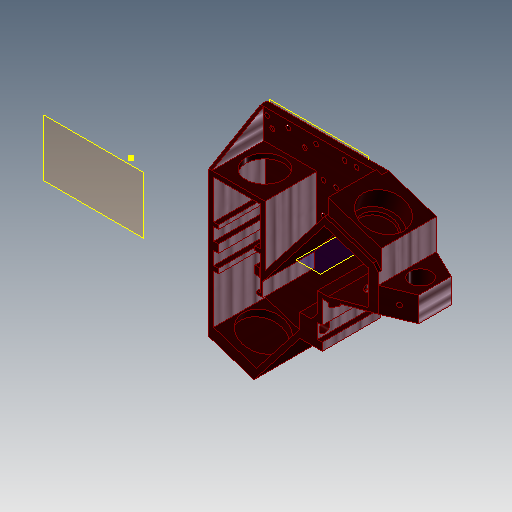
# Autodesk Inventor part: cellSTORM_v5_opticalstage
Saved by Autodesk Inventor 2019.4 (Build 234330000, 330)
## iProperties
Created: 2020-04-25
Part Number: cellSTORM_v5_opticalstage
Material: Generic
Document SubType Name: Modeling
Designer: diederichbenedict
Density: 1 g/cm^3
Appearance: Red
Author: diederichbenedict
Autodesk Inventor part; units mm, degrees
ref_plane "YZ Plane" through (0, 0, 0) normal (1, 0, 0) x (0, 1, 0)
ref_plane "XZ Plane" through (0, 0, 0) normal (0, 1, 0) x (-1, 0, 0)
ref_plane "XY Plane" through (0, 0, 0) normal (0, 0, 1) x (1, 0, 0)
ref_plane "Work Plane1" through (0, 0, 0) normal (0, 0, 1) x (1, 0, 0)
ref_plane "Work Plane2" through (79.8747, 18.953, -59.1152) normal (0, 0, 1) x (1, 0, 0)
sketch "Sketch2" plane through (79.8747, 18.953, -59.1152) normal (0, 0, 1) x (1, 0, 0)
  line L0 (-28, -14.1495) -> (28, -14.1495) projected
  line L1 (28, -14.1495) -> (28, -9.1495) projected
  line L2 (28, -9.1495) -> (22, -9.1495) projected
  line L3 (22, -9.1495) -> (22, 17.8293) projected
  line L4 (22, 17.8293) -> (-22, 17.8293) projected
  line L5 (-22, 17.8293) -> (-22, -9.1495) projected
  line L6 (-22, -9.1495) -> (-28, -9.1495) projected
  line L7 (-28, -9.1495) -> (-28, -14.1495) projected
  line L8 (-28, -14.1495) -> (-32, -14.1495)
  line L9 (-28, -14.1495) -> (-24, -14.1495) construction
  line L10 (-32, -14.1495) -> (-32, -90.2028)
  line L11 (-32, -90.2028) -> (-4.0389, -99.2879)
  line L12 (-4.0389, -99.2879) -> (46.0734, -35.147)
  line L13 (46.0734, -35.147) -> (72.5683, -35.147)
  line L14 (72.5683, -35.147) -> (72.5683, 8.2211)
  line L15 (72.5683, 8.2211) -> (42.9972, 17.8293)
  line L16 (42.9972, 17.8293) -> (22, 17.8293)
  line L17 (-28.3388, -86.702) -> (-4.6575, -94.3965) projected
  line L18 (-4.3425, -94.236) -> (-28.4993, -86.387) projected
  line L19 (45.4114, 13.8905) -> (69.5683, 6.0415) projected
  line L20 (-27.6911, -86.6496) -> (-26.7997, -83.9062)
  line L21 (-3.5343, -94.4986) -> (-2.6429, -91.7552)
  line L22 (53.5499, -4.91) -> (-11.1218, -87.6859)
  line L23 (-22, 17.8293) -> (-32, 17.8293)
  line L24 (-32, 17.8293) -> (-32, -14.1495)
  point P0 (-79.8747, -18.953)
  point P1 (-26.7997, -83.9062)
  point P2 (-2.6429, -91.7552)
  dimension "d0" = 4
  dimension "d1" = 180
  dimension "d2" = 3
  dimension "d3" = 3
  dimension "d4" = 3
  dimension "d5" = 1
  constraints: 28 end point, 7 parallel, 3 collinear, 3 horizontal, 1 perpendicular, 7 other
  measures "d0" distance of L0.start L8.end
  measures "d1" angle of L8 L9
  measures "d2" distance between parallel lines of L19 L15
  measures "d3" distance from line of L19.end L14
  measures "d4" distance from line of L20 L10.end
  measures "d5" distance from line of L11.end L21
extrude "Extrusion1" add sketch "Sketch2" along normal blind 4
sketch "Sketch3" plane through (79.8747, 18.953, -55.1152) normal (0, 0, 1) x (1, 0, 0)
  line L0 (42.9972, 17.8293) -> (-32, 17.8293) projected
  line L1 (-32, 17.8293) -> (-32, -90.2028) projected
  line L2 (-32, -90.2028) -> (-4.0389, -99.2879) projected
  line L3 (-4.0389, -99.2879) -> (46.0734, -35.147) projected
  line L4 (46.0734, -35.147) -> (72.5683, -35.147) projected
  line L5 (72.5683, -35.147) -> (72.5683, 8.2211) projected
  line L6 (72.5683, 8.2211) -> (42.9972, 17.8293) projected
  line L7 (-27.1008, 14.8293) -> (42.5221, 14.8293)
  line L8 (42.5221, 14.8293) -> (69.5683, 6.0415)
  line L9 (66.4162, -32.147) -> (35.0734, -32.147)
  line L10 (-2.489, -92.4313) -> (-29, -83.8173)
  line L11 (-28.6512, -0.5207) -> (-0.8512, -0.5207) projected
  line L12 (-29, -3.5207) -> (-27.1008, -3.5207)
  line L13 (2.7488, -0.5207) -> (2.7488, -4.5207)
  line L14 (-0.2512, -3.5207) -> (-29, -3.5207)
  line L15 (-32, 17.8293) -> (-32, -90.2028) projected
  line L16 (-12.2512, -81.0102) -> (-12.2512, 6.7293) construction
  line L17 (52.4205, 1.7657) -> (-12.2512, -81.0102) construction
  line L18 (2.7488, -4.5207) -> (2.7488, -37.447)
  line L19 (2.7488, -37.447) -> (39.6078, 9.7303)
  line L20 (43.8723, 8.3447) -> (67.5537, 0.6501) projected
  line L21 (-0.2512, -3.5207) -> (-0.2512, -46.1597)
  line L22 (-0.2512, -46.1597) -> (39.3735, 4.5576)
  line L23 (39.3735, 4.5576) -> (66.4162, -4.2291)
  line L24 (39.6078, 9.7303) -> (69.5683, -0.0045)
  line L25 (-29, -83.8173) -> (-29, -3.5207)
  line L26 (69.5683, -0.0045) -> (72.5683, -3.7292)
  line L27 (72.5683, -35.147) -> (72.5683, 8.2211) projected
  line L28 (66.0925, 1.3476) -> (69.5683, -0.0045)
  line L29 (66.4162, -4.2291) -> (66.4162, -32.147)
  line L30 (-3.2512, -3.2707) -> (-3.2512, -19.4707) construction
  line L31 (-29.0012, -37.7707) -> (-0.5012, -37.7707) projected
  line L32 (-0.5012, -37.7707) -> (-0.5012, -30.5207) projected
  line L33 (-29.0012, -30.5207) -> (-0.5012, -30.5207) projected
  line L34 (-29.0012, -37.7707) -> (-29.0012, -30.5207) projected
  line L35 (-29.0012, -37.7707) -> (-0.5012, -37.7707) construction
  line L36 (-29, -37.7707) -> (-26, -37.7707) construction
  line L37 (-26, -37.7707) -> (-26, -42.7707) construction
  line L38 (-26, -42.7707) -> (-29, -42.7707) construction
  line L39 (-29, -42.7707) -> (-29, -37.7707) construction
  line L40 (-29, -42.7707) -> (-26, -42.7707)
  line L41 (-26, -42.7707) -> (-26, -37.7707)
  line L42 (-26, -37.7707) -> (-29, -37.7707)
  line L43 (-29, -37.7707) -> (-29, -42.7707)
  line L44 (-0.5012, -37.7707) -> (-3.5012, -37.7707)
  line L45 (-3.5012, -37.7707) -> (-3.5012, -42.7707)
  line L46 (-3.5012, -42.7707) -> (-0.5012, -42.7707)
  line L47 (-0.5012, -42.7707) -> (-0.5012, -37.7707)
  line L48 (-29, -27.5207) -> (-26, -27.5207)
  line L49 (-26, -27.5207) -> (-26, -30.0207)
  line L50 (-26, -30.0207) -> (-29, -30.0207)
  line L51 (-29, -30.0207) -> (-29, -27.5207)
  line L52 (-0.2512, -27.5207) -> (-3.5012, -27.5207)
  line L53 (-3.5012, -27.5207) -> (-3.5012, -30.0207)
  line L54 (-3.5012, -30.0207) -> (-0.2512, -30.0207)
  line L55 (-0.2512, -30.0207) -> (-0.2512, -27.5207)
  line L56 (-4.0389, -99.2879) -> (46.0734, -35.147) projected
  line L57 (46.0734, -35.147) -> (72.5683, -35.147) projected
  line L58 (39.6078, 9.7303) -> (45.1198, 17.1396)
  line L59 (72.5683, 8.2211) -> (42.9972, 17.8293) projected
  line L60 (72.5683, -3.7292) -> (72.5683, 8.2211)
  line L61 (72.5683, 8.2211) -> (45.1198, 17.1396)
  line L62 (2.7488, -0.5207) -> (-32, -0.5207)
  line L63 (35.0734, -32.147) -> (35.0734, -44.3536)
  line L64 (35.0734, -44.3536) -> (-2.489, -92.4313)
  line L65 (38.0734, -45.3866) -> (38.0734, -35.147)
  line L66 (38.0734, -35.147) -> (46.0734, -35.147)
  line L67 (38.0734, -45.3866) -> (42.0734, -45.3866)
  line L68 (42.0734, -45.3866) -> (42.0734, -48.3866)
  line L69 (42.0734, -48.3866) -> (35.7295, -48.3866)
  point P0 (-79.8747, -18.953)
  point P1 (-0.8512, -0.5207)
  point P2 (-32, -3.2707)
  dimension "d10" = 4
  dimension "d11" = 3
  dimension "d13" = 3
  dimension "d16" = 12
  dimension "d17" = 3
  dimension "d18" = 3
  dimension "d19" = 5
  dimension "d20" = 3
  dimension "d21" = 2.5
  dimension "d22" = 0.5
  dimension "d23" = 3
  dimension "d24" = 7
  dimension "d25" = 3
  dimension "d47" = 3
  dimension "d48" = 3
  dimension "d49" = 3
  dimension "d50" = 8
  dimension "d51" = 3
  dimension "d66" = 4
  constraints: 100 end point, 17 parallel, 15 point on line, 10 perpendicular, 8 horizontal, 6 vertical, 2 collinear, 13 other
  measures "d10" distance of L13.start L13.end
  measures "d13" distance between parallel lines of L22 L19
  measures "d16" distance between parallel lines of L22 L17
  measures "d18" distance of L37.end L38.end
  measures "d19" distance of L36.end L37.end
  measures "d20" distance of L46.end L45.end
  measures "d21" distance of L48.end L49.end
  measures "d22" distance between parallel lines of L33 L50
  measures "d24" distance between parallel lines of L2 L10
  measures "d25" distance between parallel lines of L25 L1
  measures "d47" distance between parallel lines of L9 L4
  measures "d48" distance between parallel lines of L64 L3
  measures "d49" distance between parallel lines of L63 L65
  measures "d50" distance from line of L3.end L65
  measures "d51" distance of L67.end L68.end
  measures "d66" distance between parallel lines of L68 L65
extrude "Extrusion2" add sketch "Sketch3" along normal blind 32 contours L62 L11 L13 L18 L19 L24 L20 L26 L5 L4 L66 L65 L3 L2 L1 | L54 L53 L52 L21 | L25 L31 L41 L40 | L25 L48 L49 L50 | L31 L47 L46 L45
ref_plane "Work Plane3" through (51.6835, -64.2382, -58.0722) normal (0.309017, 0.9510565, 0) x (-0.6726294, 0.2185505, 0.7069691)
ref_plane "Work Plane4" through (49.8294, -69.9446, -58.0722) normal (-0.309017, -0.9510565, 0) x (0.6723676, -0.2184655, 0.7072444)
sketch "Sketch7" plane through (50.8747, -64.8644, -23.1152) normal (0.309017, 0.9510565, 0) x (0.9510565, -0.309017, 0)
  circle A0 centre (13.9703, 17.35) radius 12.7 projected
  circle A1 centre (13.9703, 17.35) radius 13
  point P0 (-68.4289, -23.1152)
  dimension "d33" = 26
  constraints: 1 centre point, 1 coincident
  measures "d33" diameter of A1
extrude "Extrusion5" cut sketch "Sketch7" against normal up to surface (6 mm away) from surface at 0.8454 contours A0 | A1
sketch "Sketch8" plane through (79.8747, 18.953, -55.1152) normal (0, 0, 1) x (1, 0, 0)
  line L0 (-32, -90.2028) -> (-4.0389, -99.2879) projected
  line L1 (72.5683, -35.147) -> (72.5683, -3.7292) projected
  line L2 (69.5683, -0.0045) -> (39.6078, 9.7303) projected
  line L3 (39.6078, 9.7303) -> (2.7488, -37.447) projected
  line L4 (2.7488, -37.447) -> (2.7488, -0.5207) projected
  line L5 (-32, -0.5207) -> (-32, -90.2028) projected
  line L6 (-29, -30.5207) -> (-29, -30.0207) projected
  line L7 (-29, -30.0207) -> (-26, -30.0207) projected
  line L8 (-26, -30.0207) -> (-26, -27.5207) projected
  line L9 (-26, -27.5207) -> (-29, -27.5207) projected
  line L10 (-29, -27.5207) -> (-29, -3.5207) projected
  line L11 (-29, -3.5207) -> (-0.2512, -3.5207) projected
  line L12 (-0.2512, -27.5207) -> (-3.5012, -27.5207) projected
  line L13 (-3.5012, -27.5207) -> (-3.5012, -30.0207) projected
  line L14 (-3.5012, -30.0207) -> (-0.2512, -30.0207) projected
  line L15 (-0.5012, -37.7707) -> (-3.5012, -37.7707) projected
  line L16 (-3.5012, -37.7707) -> (-3.5012, -42.7707) projected
  line L17 (-3.5012, -42.7707) -> (-0.5012, -42.7707) projected
  line L18 (-0.2512, -46.1597) -> (39.3735, 4.5576) projected
  line L19 (39.3735, 4.5576) -> (66.4162, -4.2291) projected
  line L20 (66.4162, -4.2291) -> (66.4162, -32.147) projected
  line L21 (66.4162, -32.147) -> (35.0734, -32.147) projected
  line L22 (-2.489, -92.4313) -> (-29, -83.8173) projected
  line L23 (-29, -83.8173) -> (-29, -42.7707) projected
  line L24 (-29, -42.7707) -> (-26, -42.7707) projected
  line L25 (-26, -42.7707) -> (-26, -37.7707) projected
  line L26 (-26, -37.7707) -> (-29.0012, -37.7707) projected
  line L27 (-29.0012, -37.7707) -> (-29.0012, -30.5207) projected
  line L28 (-29.0012, -30.5207) -> (-29, -30.5207) projected
  line L29 (39.6078, 9.7303) -> (73.3765, -1.2418) projected
  line L30 (39.6078, 9.7303) -> (39.6078, 18.9306)
  line L31 (72.5683, 8.2211) -> (42.9972, 17.8293) projected
  line L32 (39.6078, 18.9306) -> (72.5683, 8.2211)
  line L33 (72.5683, -3.7292) -> (72.5683, 8.2211) projected
  line L34 (72.5683, 8.2211) -> (72.5683, -3.7292)
  line L35 (72.5683, -3.7292) -> (69.5683, -0.0045) projected
  line L36 (-4.0389, -99.2879) -> (38.0734, -45.3866) projected
  line L37 (38.0734, -35.147) -> (72.5683, -35.147) projected
  line L38 (2.7488, -0.5207) -> (-32, -0.5207) projected
  line L39 (35.0734, -32.147) -> (35.0734, -44.3536) projected
  line L40 (35.0734, -44.3536) -> (-2.489, -92.4313) projected
  line L41 (38.0734, -45.3866) -> (38.0734, -35.147) projected
  line L42 (-0.5012, -42.7707) -> (-0.5012, -37.7707) projected
  line L43 (-0.2512, -3.5207) -> (-0.2512, -27.5207) projected
  line L44 (-0.2512, -30.0207) -> (-0.2512, -46.1597) projected
  point P0 (-79.8747, -18.953)
  constraints: 6 end point, 2 vertical, 1 collinear, 1 point on line
extrude "Extrusion6" add sketch "Sketch8" along normal blind 30 contours L30 L32 L31 L33 L29 L2 | L35 L29 L33
sketch "Sketch9" plane through (122.8719, 36.7823, -55.1152) normal (0.309017, 0.9510565, 0) x (0.9510565, -0.309017, 0)
  circle A0 centre (16.2132, -14.65) radius 12.7 projected
  circle A1 centre (16.2132, -14.65) radius 13
  point P0 (-105.4918, -55.1152)
  dimension "d38" = 26
  constraints: 1 centre point, 1 coincident
  measures "d38" diameter of A1
ref_plane "Work Plane5" through (122.0405, 25.1021, -58.0722) normal (-0.309017, -0.9510565, 0) x (0.6723676, -0.2184655, 0.7072444)
extrude "Extrusion7" cut sketch "Sketch9" against normal up to surface (11.3654 mm away) contours A0 | A1
sketch "Sketch10" plane through (134.7795, 20.963, -40.4652) normal (0.309017, 0.9510565, 0) x (0.9510565, -0.309017, 0)
  circle A0 centre (0, 0) radius 12.45 projected
  circle A1 centre (0, 0) radius 10.2077
  point P0 (-121.705, -40.4652)
  constraints: 1 centre point, 1 coincident
extrude "Extrusion8" cut sketch "Sketch10" against normal blind 20 contours A1
sketch "Sketch11" plane through (47.8747, 18.4323, -55.1152) normal (0, 1, 0) x (1, 0, 0)
  circle A0 centre (17.2488, -14.65) radius 13.9 projected
  circle A1 centre (17.2488, -14.65) radius 11.75
  point P0 (-47.8747, -55.1152)
  dimension "d43" = 23.5
  constraints: 1 centre point, 1 coincident
  measures "d43" diameter of A1
extrude "Extrusion9" cut sketch "Sketch11" along normal mid plane 20 contours A1
sketch "Sketch12" plane through (125.9481, -16.1941, -59.1152) normal (0, -1, 0) x (1, 0, 0)
  circle A0 centre (9.9765, 18.65) radius 7 projected
  circle A1 centre (9.9765, 18.65) radius 10
  point P0 (-125.9481, 59.1152)
  dimension "d52" = 20
  constraints: 1 centre point, 1 coincident
  measures "d52" diameter of A1
extrude "Extrusion10" cut sketch "Sketch12" against normal up to surface contours A0 | A1 surface through (146.2909, 14.7238, -55.1152) normal (0.309017, 0.9510565, 0)
sketch "Sketch13" plane through (79.8747, 18.953, -55.1152) normal (0, 0, 1) x (1, 0, 0)
  line L0 (39.6078, 9.7303) -> (39.6078, 17.8293) construction
  line L1 (39.6078, 17.8293) -> (-32, 17.8293) construction
  line L2 (-32, 17.8293) -> (-32, -0.5207) construction
  line L3 (-32, -0.5207) -> (2.7488, -0.5207) construction
  line L4 (2.7488, -0.5207) -> (2.7488, -37.447) construction
  line L5 (2.7488, -37.447) -> (39.6078, 9.7303) construction
  line L6 (-28, 13.8293) -> (35.6078, 13.8293) construction
  line L7 (35.6078, 13.8293) -> (35.6078, 11.1076) construction
  line L8 (35.6078, 11.1076) -> (6.7488, -25.8302) construction
  line L9 (6.7488, -25.8302) -> (6.7488, 3.4793) construction
  line L10 (6.7488, 3.4793) -> (-28, 3.4793) construction
  line L11 (-28, 3.4793) -> (-28, 13.8293) construction
  line L12 (-29, -27.5207) -> (-29, -3.5207) construction
  line L13 (-0.2512, -3.5207) -> (-0.2512, -27.5207) projected
  point P0 (-79.8747, -18.953)
  point P1 (-28, 13.8795)
  point P2 (2.2283, 13.8293)
  point P3 (27.2605, 13.8293)
  point P4 (24.4005, -3.237)
  point P5 (6.7488, -3.2707)
  point P6 (-4.2512, -23.8533)
  point P7 (-25, -23.8533)
  point P8 (-15.0063, 13.8293)
  point P9 (19.8117, 13.8293)
  point P10 (14.5771, -3.2707)
  point P11 (6.7488, -22.2564)
  dimension "d55" = 4
  dimension "d56" = 4
  dimension "d65" = 4
  constraints: 12 end point, 8 point on line, 1 coincident, 5 other
  measures "d55" distance between parallel lines of L1 L6
  measures "d56" distance from line of point (-25, -23.853) L12
  measures "d65" distance from line of L13 point (-4.251, -23.853)
hole "Hole1" at (51.8747, 32.8325, -55.1152) at (82.103, 32.7823, -55.1152) at (107.1351, 32.7823, -55.1152) at (104.2752, 15.716, -55.1152) at (86.6235, 15.6823, -55.1152) at (75.6235, -4.9003, -55.1152) at (54.8747, -4.9003, -55.1152) at (86.6235, -3.3034, -55.1152) at (94.4518, 15.6823, -55.1152) at (99.6864, 32.7823, -55.1152) at (64.8684, 32.7823, -55.1152) direction (0, 0, -1) diameter 2.9 depth 8 tip angle 118
sketch "Sketch14" plane through (79.8747, 18.953, -23.1152) normal (0, 0, 1) x (1, 0, 0)
  line L0 (39.6078, 9.7303) -> (2.7488, -37.447) projected
  line L1 (2.7488, -37.447) -> (2.7488, -0.5207) projected
  line L2 (2.7488, -0.5207) -> (-32, -0.5207) projected
  line L3 (-32, -0.5207) -> (-32, -90.2028) projected
  line L4 (-32, -90.2028) -> (-4.0389, -99.2879) projected
  line L5 (-4.0389, -99.2879) -> (38.0734, -45.3866) projected
  line L6 (38.0734, -45.3866) -> (38.0734, -35.147) projected
  line L7 (38.0734, -35.147) -> (72.5683, -35.147) projected
  line L8 (72.5683, -35.147) -> (72.5683, -3.7292) projected
  line L9 (-29, -30.5207) -> (-29, -30.0207) projected
  line L10 (-29, -30.0207) -> (-26, -30.0207) projected
  line L11 (-26, -30.0207) -> (-26, -27.5207) projected
  line L12 (-26, -27.5207) -> (-29, -27.5207) projected
  line L13 (-29, -27.5207) -> (-29, -3.5207) projected
  line L14 (-29, -3.5207) -> (-0.2512, -3.5207) projected
  line L15 (-0.2512, -3.5207) -> (-0.2512, -27.5207) projected
  line L16 (-0.2512, -27.5207) -> (-3.5012, -27.5207) projected
  line L17 (-3.5012, -27.5207) -> (-3.5012, -30.0207) projected
  line L18 (-3.5012, -30.0207) -> (-0.2512, -30.0207) projected
  line L19 (-0.2512, -30.0207) -> (-0.2512, -46.1597) projected
  line L20 (-0.5012, -37.7707) -> (-3.5012, -37.7707) projected
  line L21 (-3.5012, -37.7707) -> (-3.5012, -42.7707) projected
  line L22 (-3.5012, -42.7707) -> (-0.5012, -42.7707) projected
  line L23 (-0.2512, -46.1597) -> (39.3735, 4.5576) projected
  line L24 (39.3735, 4.5576) -> (66.4162, -4.2291) projected
  line L25 (66.4162, -4.2291) -> (66.4162, -32.147) projected
  line L26 (66.4162, -32.147) -> (35.0734, -32.147) projected
  line L27 (35.0734, -32.147) -> (35.0734, -44.3536) projected
  line L28 (35.0734, -44.3536) -> (-2.489, -92.4313) projected
  line L29 (-2.489, -92.4313) -> (-29, -83.8173) projected
  line L30 (-29, -83.8173) -> (-29, -42.7707) projected
  line L31 (-29, -42.7707) -> (-26, -42.7707) projected
  line L32 (-26, -42.7707) -> (-26, -37.7707) projected
  line L33 (-26, -37.7707) -> (-29.0012, -37.7707) projected
  line L34 (-29.0012, -37.7707) -> (-29.0012, -30.5207) projected
  line L35 (-29.0012, -30.5207) -> (-29, -30.5207) projected
  line L36 (-4.0389, -99.2879) -> (46.0734, -35.147) projected
  line L37 (35.0734, -49.2264) -> (35.0734, -58.2264)
  line L38 (35.0734, -58.2264) -> (28.0418, -58.2264)
  line L39 (28.0418, -58.2264) -> (35.0734, -49.2264)
  line L40 (-4.0389, -99.2879) -> (38.0734, -45.3866) projected
  line L41 (72.5683, -3.7292) -> (69.5683, -0.0045) projected
  line L42 (69.5683, -0.0045) -> (39.6078, 9.7303) projected
  line L43 (35.0734, -44.3536) -> (-2.489, -92.4313) projected
  line L44 (31.3468, -49.1234) -> (24.2348, -49.1234)
  line L45 (24.2348, -49.1234) -> (24.2348, -58.2264)
  line L46 (24.2348, -58.2264) -> (31.3468, -49.1234)
  line L47 (24.2348, -63.0992) -> (38.0734, -63.0992)
  line L48 (38.0734, -63.0992) -> (38.0734, -58.2264)
  line L49 (38.0734, -58.2264) -> (35.0734, -58.2264)
  line L50 (38.0734, -45.3866) -> (38.0734, -49.2264)
  line L51 (38.0734, -49.2264) -> (35.0734, -49.2264)
  line L52 (-0.5012, -42.7707) -> (-0.5012, -37.7707) projected
  point P0 (-79.8747, -18.953)
  dimension "d67" = 9
  dimension "d68" = 0
  constraints: 22 end point, 10 point on line, 5 perpendicular, 2 horizontal, 1 collinear, 1 vertical
  measures "d67" distance of L37.start L37.end
  measures "d68" distance between parallel lines of L37 L27
extrude "Extrusion11" add sketch "Sketch14" against normal up to surface (36 mm away) contours L50 L51 L5 | L5 L38 L49 L48 L47 | L37 L38 L5 | L45 L44 L28
sketch "Sketch15" plane through (114.9481, -39.2734, -23.1152) normal (1, 0, 0) x (0, 0, -1)
  line L0 (0, 0) -> (0, 9) projected
  circle A0 centre (4.35, 4.5) radius 1.4
  circle A1 centre (30.35, 4.5) radius 1.4
  line L1 (4.35, 11.0794) -> (4.35, -28.9206)
  line L2 (30.35, 11.0794) -> (30.35, -28.9206)
  line L3 (0, 0) -> (36, 0) projected
  line L4 (0, 9) -> (36, 9) projected
  line L5 (36, 9) -> (36, 0) projected
  point P0 (-23.1152, 39.2734)
  dimension "d71" = 2.8
  dimension "d72" = 2.8
  constraints: 4 end point, 2 centre point, 2 point on line, 2 vertical, 4 other
  measures "d71" diameter of A0
  measures "d72" diameter of A1
hole "Hole2" at (114.9481, -34.7734, -27.4652) at (114.9481, -34.7734, -53.4652) direction (-1, 0, 0) diameter 6.756 depth 12 tip angle 118 clearance for "Hex Head Bolt" size "1/4" standard "Ansi Unified Screw Threads"
sketch "Sketch16" plane through (79.8747, 18.953, -23.1152) normal (0, 0, 1) x (1, 0, 0)
  line L0 (46.0734, -35.147) -> (38.0734, -35.147) projected
  line L1 (38.0734, -35.147) -> (38.0734, -45.3866) projected
  line L2 (38.0734, -45.3866) -> (46.0734, -35.147) projected
  line L3 (38.0734, -35.147) -> (72.5683, -25.9042)
  line L4 (72.5683, -35.147) -> (72.5683, 8.2211) projected
  line L5 (38.0734, -35.147) -> (73.7851, -35.147) construction
  line L6 (72.5683, -25.9042) -> (72.5683, -35.147)
  line L7 (72.5683, -35.147) -> (46.0734, -35.147)
  line L8 (72.5683, -35.147) -> (38.0734, -45.3866)
  point P0 (-79.8747, -18.953)
  dimension "d84" = 15
  constraints: 10 end point, 1 collinear, 1 equal length, 1 horizontal, 1 perpendicular, 1 point on line
  measures "d84" angle of L5 L3
extrude "Extrusion13" cut sketch "Sketch16" against normal through all
sketch "Sketch17" plane through (79.8747, 18.953, -23.1152) normal (0, 0, 1) x (1, 0, 0)
  point P0 (-79.8747, -18.953)
sketch "Sketch18" plane through (79.8747, 18.953, -23.1152) normal (0, 0, 1) x (1, 0, 0)
  line L0 (66.4162, -27.5526) -> (72.5683, -25.9042) projected
  line L1 (72.5683, -25.9042) -> (72.5683, -3.7292) projected
  line L2 (72.5683, -3.7292) -> (69.5683, -0.0045) projected
  line L3 (69.5683, -0.0045) -> (39.6078, 9.7303) projected
  line L4 (39.6078, 9.7303) -> (2.7488, -37.447) projected
  line L5 (2.7488, -37.447) -> (2.7488, -0.5207) projected
  line L6 (2.7488, -0.5207) -> (-32, -0.5207) projected
  line L7 (-32, -0.5207) -> (-32, -90.2028) projected
  line L8 (-32, -90.2028) -> (-4.0389, -99.2879) projected
  line L9 (-4.0389, -99.2879) -> (24.2348, -63.0992) projected
  line L10 (24.2348, -63.0992) -> (38.0734, -63.0992) projected
  line L11 (38.0734, -63.0992) -> (38.0734, -58.2264) projected
  line L12 (38.0734, -58.2264) -> (35.0734, -58.2264) projected
  line L13 (35.0734, -58.2264) -> (35.0734, -49.2264) projected
  line L14 (35.0734, -49.2264) -> (38.0734, -49.2264) projected
  line L15 (38.0734, -49.2264) -> (38.0734, -35.147) projected
  line L16 (38.0734, -35.147) -> (49.2696, -32.147) projected
  line L17 (49.2696, -32.147) -> (35.0734, -32.147) projected
  line L18 (35.0734, -32.147) -> (35.0734, -44.3536) projected
  line L19 (35.0734, -44.3536) -> (31.3468, -49.1234) projected
  line L20 (31.3468, -49.1234) -> (24.2348, -49.1234) projected
  line L21 (24.2348, -49.1234) -> (24.2348, -58.2264) projected
  line L22 (24.2348, -58.2264) -> (-2.489, -92.4313) projected
  line L23 (-2.489, -92.4313) -> (-29, -83.8173) projected
  line L24 (-29, -83.8173) -> (-29, -42.7707) projected
  line L25 (-29, -42.7707) -> (-26, -42.7707) projected
  line L26 (-26, -42.7707) -> (-26, -37.7707) projected
  line L27 (-26, -37.7707) -> (-29.0012, -37.7707) projected
  line L28 (-29.0012, -37.7707) -> (-29.0012, -30.5207) projected
  line L29 (-29.0012, -30.5207) -> (-29, -30.5207) projected
  line L30 (-29, -30.5207) -> (-29, -30.0207) projected
  line L31 (-29, -30.0207) -> (-26, -30.0207) projected
  line L32 (-26, -30.0207) -> (-26, -27.5207) projected
  line L33 (-26, -27.5207) -> (-29, -27.5207) projected
  line L34 (-29, -27.5207) -> (-29, -3.5207) projected
  line L35 (-29, -3.5207) -> (-0.2512, -3.5207) projected
  line L36 (-0.2512, -3.5207) -> (-0.2512, -27.5207) projected
  line L37 (-0.2512, -27.5207) -> (-3.5012, -27.5207) projected
  line L38 (-3.5012, -27.5207) -> (-3.5012, -30.0207) projected
  line L39 (-3.5012, -30.0207) -> (-0.2512, -30.0207) projected
  line L40 (-0.2512, -30.0207) -> (-0.2512, -46.1597) projected
  line L41 (-0.5012, -37.7707) -> (-3.5012, -37.7707) projected
  line L42 (-3.5012, -37.7707) -> (-3.5012, -42.7707) projected
  line L43 (-3.5012, -42.7707) -> (-0.5012, -42.7707) projected
  line L44 (-0.2512, -46.1597) -> (39.3735, 4.5576) projected
  line L45 (39.3735, 4.5576) -> (66.4162, -4.2291) projected
  line L46 (66.4162, -4.2291) -> (66.4162, -27.5526) projected
  line L47 (38.0734, -35.147) -> (49.2696, -32.147) projected
  line L48 (38.0734, -35.147) -> (41.7751, -35.147)
  line L49 (41.7751, -35.147) -> (41.7751, -37.2752)
  line L50 (41.7751, -37.2752) -> (47.3264, -37.2752)
  line L51 (47.3264, -37.2752) -> (49.2696, -32.147)
  line L52 (49.2696, -32.147) -> (38.0734, -35.147)
  line L53 (-0.5012, -42.7707) -> (-0.5012, -37.7707) projected
  point P0 (-79.8747, -18.953)
  constraints: 10 end point, 2 perpendicular, 1 collinear, 1 horizontal
extrude "Extrusion14" add sketch "Sketch18" against normal up to surface (36 mm away) contours L16 L51 L50 L49 L48
sketch "Sketch19" plane through (152.443, -6.9512, -59.1152) normal (0.258819, -0.9659258, 0) x (0.9659258, 0.258819, 0)
  line L0 (-24.1206, 4) -> (-24.1206, 0) projected
  line L1 (0, 0) -> (-24.1206, 0) projected
  line L2 (0, 36) -> (0, 0) projected
  line L3 (-6.3691, 36) -> (0, 36) projected
  line L4 (-6.3691, 4) -> (-6.3691, 36) projected
  line L5 (-24.1206, 4) -> (-6.3691, 4) projected
  line L6 (-27.3248, 36) -> (-24.1206, 36) projected
  line L7 (0, 36) -> (0, 0) projected
  line L8 (0, 0) -> (-32.1686, 0)
  line L9 (-32.1686, 0) -> (-32.1686, 36)
  line L10 (-32.1686, 36) -> (0, 36)
  line L11 (0, 36) -> (0, 0)
  point P0 (-145.4495, 59.1152)
  constraints: 8 end point, 2 parallel, 1 horizontal, 1 perpendicular, 1 point on line
extrude "Extrusion15" add sketch "Sketch19" against normal blind 2
chamfer "Chamfer1" distance 4 angle 45 1 edges at (127.2011, -18.3222, -41.1152)
ref_plane "Work Plane6" through (104.1095, -1.6462, -23.1152) normal (0, -1, 0) x (1, 0, 0)
sketch "Sketch20" plane through (104.1095, -1.6462, -23.1152) normal (0, -1, 0) x (1, 0, 0)
  line L0 (48.3335, 0) -> (48.3335, -36) projected
  line L1 (48.3335, -36) -> (48.3335, -2) projected
  line L2 (48.3335, -2) -> (48.3335, 0) projected
  line L3 (57.5751, -17.35) -> (20.0551, -17.35)
  line L4 (59.3302, -3.2257) -> (59.3302, -31.4743) projected
  line L5 (53.4849, -8.4131) -> (53.4849, -26.2869) projected
  circle A0 centre (57.1891, -17.35) radius 6
  line L6 (66.0447, -27.35) -> (48.3335, -27.35)
  line L7 (48.3335, -27.35) -> (48.3335, -7.35)
  line L8 (48.3335, -7.35) -> (66.0447, -7.35)
  line L9 (66.0447, -7.35) -> (66.0447, -27.35)
  line L10 (66.0447, -27.35) -> (48.3335, -7.35) construction
  line L11 (48.3335, -27.35) -> (66.0447, -7.35) construction
  line L12 (66.0447, -7.35) -> (48.3335, 0)
  line L13 (66.0447, -27.35) -> (48.3335, -36)
  line L14 (48.3335, 0) -> (48.3335, -7.35)
  line L15 (48.3335, -36) -> (48.3335, -27.35)
  circle A1 centre (57.1891, -17.35) radius 6.335 projected
  circle A2 centre (57.1891, -17.35) radius 6.535
  point P0 (-104.1095, 23.1152)
  dimension "d95" = 12
  dimension "d96" = 20
  dimension "d103" = 0.2
  constraints: 22 end point, 2 centre point, 2 collinear, 2 horizontal, 2 midpoint, 2 parallel, 2 point on line, 1 perpendicular, 2 other
  measures "d95" diameter of A0
  measures "d96" distance of L6.end L7.end
  measures "d103" radial gap between concentric circles of A1 A2
extrude "Extrusion16" add sketch "Sketch20" along normal blind 5.3 and the other way blind 10 contours L12 L4 L8 L0 | L12 L8 L4 | L8 L4 A2 L3 L0 | L8 L9 L6 L4 A2 | L3 A2 L4 L6 L0 | L13 L4 L6 | L6 L4 L13 L0
sketch "Sketch21" plane through (104.1095, -44.1462, -23.1152) normal (0, -1, 0) x (1, 0, 0)
  circle A0 centre (31.8151, -17.35) radius 7 projected
  point P0 (-104.1095, 23.1152)
extrude "Extrusion17" cut sketch "Sketch21" against normal blind 50
sketch "Sketch22" plane through (47.8747, -71.2498, -59.1152) normal (-1, 0, 0) x (0, 0, 1)
  line L0 (0, 108.0321) -> (0, 0) projected
  line L1 (0, 0) -> (36, 0) projected
  line L2 (36, 89.6821) -> (36, 0) projected
  line L3 (4, 89.6821) -> (36, 89.6821) projected
  line L4 (4, 108.0321) -> (4, 89.6821) projected
  line L5 (0, 108.0321) -> (4, 108.0321) projected
  line L6 (4, 108.0321) -> (4, 109.1334) projected
  line L7 (4, 89.6821) -> (36, 89.6821) projected
  line L8 (4, 108.0321) -> (36, 89.6821)
  line L9 (36, 89.6821) -> (4, 89.6821)
  line L10 (4, 108.0321) -> (4, 89.6821) projected
  line L11 (4, 89.6821) -> (4, 108.0321)
  point P0 (59.1152, 71.2498)
  constraints: 6 end point, 1 collinear, 1 perpendicular
extrude "Extrusion18" add sketch "Sketch22" against normal blind 2 contours L8 L3 L4
sketch "Sketch23" plane through (79.8747, 18.953, -23.1152) normal (0, 0, 1) x (1, 0, 0)
  line L0 (75.0889, -27.2492) -> (75.0889, -10.5992)
  line L1 (87.9589, -10.5992) -> (87.9589, -25.8992) projected
  circle A0 centre (81.9173, -18.2492) radius 1.4
  point P0 (-79.8747, -18.953)
  dimension "d106" = 2.8
  constraints: 2 end point, 1 centre point, 1 vertical, 2 other
  measures "d106" diameter of A0
extrude "Extrusion19" cut sketch "Sketch23" against normal through all
sketch "Sketch24" plane through (79.8747, 18.953, -55.1152) normal (0, 0, 1) x (1, 0, 0)
  line L0 (41.5421, -32.147) -> (66.4162, -25.482) projected
  line L1 (66.4162, -25.482) -> (66.4162, -4.2291) projected
  line L2 (66.4162, -4.2291) -> (39.3735, 4.5576) projected
  line L3 (39.3735, 4.5576) -> (-0.2512, -46.1597) projected
  line L4 (-0.2512, -46.1597) -> (-0.2512, -30.0207) projected
  line L5 (-0.5012, -42.7707) -> (-3.5012, -42.7707) projected
  line L6 (-3.5012, -42.7707) -> (-3.5012, -37.7707) projected
  line L7 (-3.5012, -37.7707) -> (-0.5012, -37.7707) projected
  line L8 (-0.2512, -30.0207) -> (-3.5012, -30.0207) projected
  line L9 (-3.5012, -30.0207) -> (-3.5012, -27.5207) projected
  line L10 (-3.5012, -27.5207) -> (-0.2512, -27.5207) projected
  line L11 (-0.2512, -27.5207) -> (-0.2512, -3.5207) projected
  line L12 (-0.2512, -3.5207) -> (-29, -3.5207) projected
  line L13 (-29, -3.5207) -> (-29, -27.5207) projected
  line L14 (-29, -27.5207) -> (-26, -27.5207) projected
  line L15 (-26, -27.5207) -> (-26, -30.0207) projected
  line L16 (-26, -30.0207) -> (-29, -30.0207) projected
  line L17 (-29, -30.0207) -> (-29, -30.5207) projected
  line L18 (-29, -30.5207) -> (-29.0012, -30.5207) projected
  line L19 (-29.0012, -30.5207) -> (-29.0012, -37.7707) projected
  line L20 (-29.0012, -37.7707) -> (-26, -37.7707) projected
  line L21 (-26, -37.7707) -> (-26, -42.7707) projected
  line L22 (-26, -42.7707) -> (-29, -42.7707) projected
  line L23 (-29, -42.7707) -> (-29, -83.8173) projected
  line L24 (-29, -83.8173) -> (-2.489, -92.4313) projected
  line L25 (-2.489, -92.4313) -> (24.2348, -58.2264) projected
  line L26 (24.2348, -58.2264) -> (24.2348, -56.674) projected
  line L27 (24.2348, -49.1234) -> (31.3468, -49.1234) projected
  line L28 (31.3468, -49.1234) -> (35.0734, -44.3536) projected
  line L29 (35.0734, -44.3536) -> (35.0734, -32.147) projected
  line L30 (35.0734, -32.147) -> (41.5421, -32.147) projected
  circle A0 centre (-25, -23.8533) radius 1.45 projected
  circle A1 centre (-4.2512, -23.8533) radius 1.45 projected
  line L31 (-3.5012, -37.7707) -> (-0.5012, -37.7707) projected
  line L32 (-29.2512, -29.7707) -> (-0.2512, -29.7707)
  line L33 (-0.2512, -29.7707) -> (-0.2512, -37.7707)
  line L34 (-0.2512, -37.7707) -> (-29.2512, -37.7707)
  line L35 (-29.2512, -37.7707) -> (-29.2512, -29.7707)
  line L36 (-29, -42.7707) -> (-0.2512, -42.7707)
  line L37 (-0.2512, -42.7707) -> (-0.2512, -50.7707)
  line L38 (-29, -50.7707) -> (-29, -42.7707)
  line L39 (-29, -50.7707) -> (-29, -53.7707)
  line L40 (-29, -42.7707) -> (-29, -83.8173) projected
  line L41 (-29, -53.7707) -> (-26, -53.7707)
  line L42 (-26, -53.7707) -> (-26, -50.7707)
  line L43 (-2.2512, -50.7707) -> (-2.2512, -52.7707)
  line L44 (-2.2512, -50.7707) -> (-0.2512, -50.7707) construction
  line L45 (-2.2512, -52.7707) -> (1.4643, -52.7707)
  line L46 (1.4643, -52.7707) -> (1.4643, -43.964)
  line L47 (-0.2512, -46.1597) -> (39.3735, 4.5576) projected
  line L48 (1.4643, -43.964) -> (-0.2512, -46.1597)
  line L49 (-0.2512, -46.1597) -> (-0.2512, -50.7707)
  line L50 (-0.2512, -50.7707) -> (-2.2512, -50.7707)
  line L51 (-0.2512, -50.7707) -> (-2.2512, -50.7707)
  line L52 (-26, -50.7707) -> (-29, -50.7707)
  line L53 (24.2348, -56.674) -> (23.0734, -56.674) projected
  line L54 (23.0734, -50.7788) -> (24.2348, -50.7788) projected
  line L55 (24.2348, -50.7788) -> (24.2348, -49.1234) projected
  line L56 (-0.5012, -37.7707) -> (-0.5012, -42.7707) projected
  point P0 (-79.8747, -18.953)
  dimension "d109" = 8
  dimension "d111" = 3
  dimension "d112" = 90
  dimension "d113" = 2
  dimension "d114" = 90
  constraints: 38 end point, 8 perpendicular, 5 parallel, 5 point on line, 3 horizontal, 1 collinear, 1 vertical, 1 vertical alignment
  measures "d109" distance between parallel lines of L34 L32
  measures "d111" distance of L38.start L39.end
  measures "d112" angle of L41 L39
  measures "d113" distance of L43.start L43.end
  measures "d114" angle of L43 L44
ref_plane "Work Plane7" through (47.8747, -80.3349, -23.1152) normal (0, 0, -1) x (0, 1, 0)
extrude "Extrusion20" add sketch "Sketch24" along normal up to surface (32 mm away) contours L46 L45 L43 L50 L37 L3 | L52 L42 L41 L23
sketch "Sketch25" plane through (79.8747, 18.953, -59.1152) normal (0, 0, -1) x (-1, 0, 0)
  line L0 (0.0762, 6.8793) -> (0.0762, 10.0793) projected
  line L1 (0.0762, 6.8793) -> (0.0762, 10.0793) projected
  point P0 (79.8747, -18.953)
  point P1 (4.7512, 8.4793)
  point P2 (24.7512, 8.4793)
hole "Hole3" at (55.1235, 27.4323, -59.1152) at (75.1235, 27.4323, -59.1152) direction (0, 0, 1) diameter 3 depth 12 tip angle 118 counterbore diameter 7 counterbore depth 3
body "Solid1"
